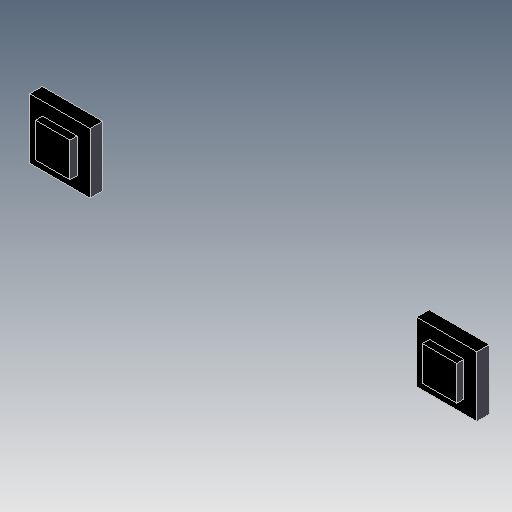
# Autodesk Inventor part: 20210330_5mmFuss_Korpus
Saved by Autodesk Inventor 2021 (Build 250183000, 183)
## iProperties
Created: 2021-03-30
Part Number: 20210330_5mmFuss_Korpus
Material: Acetal Resin, Black
Document SubType Name: Modeling
Designer: Daniel
Density: 1.425 g/cm^3
Appearance: Smooth - Black
Author: Daniel
Autodesk Inventor part; units mm, degrees
ref_plane "YZ Plane" through (0, 0, 0) normal (1, 0, 0) x (0, 1, 0)
ref_plane "XZ Plane" through (0, 0, 0) normal (0, 1, 0) x (-1, 0, 0)
ref_plane "XY Plane" through (0, 0, 0) normal (0, 0, 1) x (1, 0, 0)
sketch "Skizze1" plane through (0, 0, 0) normal (0, 0, 1) x (1, 0, 0)
  line L0 (-89, -12) -> (89, -12)
  line L1 (89, -12) -> (89, 12)
  line L2 (89, 12) -> (-89, 12)
  line L3 (-89, 12) -> (-89, -12)
  line L4 (-89, -12) -> (89, 12) construction
  line L5 (89, -12) -> (-89, 12) construction
  line L6 (65, 12) -> (65, -12)
  line L7 (-65, 12) -> (-65, -12)
  line L8 (-89, 12) -> (-65, -12) construction
  line L9 (-65, 12) -> (-89, -12) construction
  line L10 (89, 12) -> (65, -12) construction
  line L11 (65, 12) -> (89, -12) construction
  point P0 (0, 0)
  dimension "d0" = 178
  dimension "d1" = 24
  dimension "d2" = 24
  dimension "d3" = 24
  constraints: 24 end point, 4 point on line, 2 midpoint, 2 parallel, 2 perpendicular, 1 horizontal, 1 vertical
  measures "d0" distance of L1.end L2.end
  measures "d1" distance of L0.end L1.end
  measures "d2" distance between parallel lines of L1 L6
  measures "d3" distance between parallel lines of L7 L3
extrude "Extrusion1" add sketch "Skizze1" along normal blind 5
sketch "Skizze3" plane through (0, 0, 5) normal (0, 0, 1) x (1, 0, 0)
  line L0 (-89, -12) -> (89, -12)
  line L1 (89, -12) -> (89, 12)
  line L2 (89, 12) -> (-89, 12)
  line L3 (-89, 12) -> (-89, -12)
  line L4 (-89, -12) -> (89, 12) construction
  line L5 (89, -12) -> (-89, 12) construction
  line L6 (65, 12) -> (65, -12)
  line L7 (-65, 12) -> (-65, -12)
  line L8 (-89, 12) -> (-65, -12) construction
  line L9 (-65, 12) -> (-89, -12) construction
  line L10 (89, 12) -> (65, -12) construction
  line L11 (65, 12) -> (89, -12) construction
  line L12 (70.15, -6.85) -> (83.85, -6.85)
  line L13 (83.85, -6.85) -> (83.85, 6.85)
  line L14 (83.85, 6.85) -> (70.15, 6.85)
  line L15 (70.15, 6.85) -> (70.15, -6.85)
  line L16 (70.15, -6.85) -> (83.85, 6.85) construction
  line L17 (83.85, -6.85) -> (70.15, 6.85) construction
  line L18 (-83.85, -6.85) -> (-70.15, -6.85)
  line L19 (-70.15, -6.85) -> (-70.15, 6.85)
  line L20 (-70.15, 6.85) -> (-83.85, 6.85)
  line L21 (-83.85, 6.85) -> (-83.85, -6.85)
  line L22 (-83.85, -6.85) -> (-70.15, 6.85) construction
  line L23 (-70.15, -6.85) -> (-83.85, 6.85) construction
  point P0 (0, 0)
  point P1 (0, 0)
  point P2 (77, 0)
  point P3 (-77, 0)
  dimension "d10" = 178
  dimension "d11" = 24
  dimension "d12" = 24
  dimension "d13" = 24
  dimension "d14" = 13.7
  dimension "d15" = 13.7
  constraints: 48 end point, 8 midpoint, 6 parallel, 6 point on line, 4 perpendicular, 3 horizontal, 1 vertical
  measures "d10" distance of L1.end L2.end
  measures "d11" distance of L0.end L1.end
  measures "d12" distance between parallel lines of L1 L6
  measures "d13" distance between parallel lines of L7 L3
  measures "d14" distance of L13.end L14.end
  measures "d15" distance of L19.end L20.end
extrude "Extrusion2" add sketch "Skizze3" along normal blind 2.85 contours L15 L14 L13 L12 | L21 L20 L19 L18
sketch "Skizze4" plane through (0, 0, 0) normal (0, 0, -1) x (-1, 0, 0)
  line L0 (-89, -12) -> (89, -12)
  line L1 (89, -12) -> (89, 12)
  line L2 (89, 12) -> (-89, 12)
  line L3 (-89, 12) -> (-89, -12)
  line L4 (-89, -12) -> (89, 12) construction
  line L5 (89, -12) -> (-89, 12) construction
  line L6 (65, 12) -> (65, -12)
  line L7 (-65, 12) -> (-65, -12)
  line L8 (-89, 12) -> (-65, -12) construction
  line L9 (-65, 12) -> (-89, -12) construction
  line L10 (89, 12) -> (65, -12) construction
  line L11 (65, 12) -> (89, -12) construction
  line L12 (70, -7) -> (84, -7)
  line L13 (84, -7) -> (84, 7)
  line L14 (84, 7) -> (70, 7)
  line L15 (70, 7) -> (70, -7)
  line L16 (70, -7) -> (84, 7) construction
  line L17 (84, -7) -> (70, 7) construction
  line L18 (-84, -7) -> (-70, -7)
  line L19 (-70, -7) -> (-70, 7)
  line L20 (-70, 7) -> (-84, 7)
  line L21 (-84, 7) -> (-84, -7)
  line L22 (-84, -7) -> (-70, 7) construction
  line L23 (-70, -7) -> (-84, 7) construction
  point P0 (0, 0)
  point P1 (0, 0)
  point P2 (0, 0)
  point P3 (77, 0)
  point P4 (-77, 0)
  dimension "d18" = 178
  dimension "d19" = 24
  dimension "d20" = 24
  dimension "d21" = 24
  dimension "d22" = 14
  dimension "d23" = 14
  constraints: 48 end point, 8 midpoint, 6 parallel, 6 point on line, 4 perpendicular, 3 horizontal, 1 vertical
  measures "d18" distance of L1.end L2.end
  measures "d19" distance of L1.start L1.end
  measures "d20" distance between parallel lines of L1 L6
  measures "d21" distance between parallel lines of L7 L3
  measures "d22" distance of L14.start L14.end
  measures "d23" distance of L19.end L20.end
extrude "Extrusion3" cut sketch "Skizze4" against normal blind 3 contours L15 L14 L13 L12 | L21 L20 L19 L18
sketch "Skizze5" plane through (0, 0, 5) normal (0, 0, 1) x (1, 0, 0)
  line L0 (-89, 12) -> (-89, -12) projected
  line L1 (-89, -12) -> (89, -12) projected
  line L2 (-89, 12) -> (-65, 12)
  line L3 (-65, 12) -> (-65, -12)
  line L4 (-65, -12) -> (-89, -12)
  line L5 (-89, -12) -> (-89, 12)
  line L6 (89, -12) -> (89, 12) projected
  line L7 (89, 12) -> (65, 12)
  line L8 (65, 12) -> (65, -12)
  line L9 (65, -12) -> (89, -12)
  line L10 (89, -12) -> (89, 12)
  line L11 (-65, 12) -> (65, 12)
  line L12 (65, 12) -> (65, -12)
  line L13 (65, -12) -> (-65, -12)
  line L14 (-65, -12) -> (-65, 12)
  point P0 (0, 0)
  point P1 (65, -12)
  dimension "d26" = 24
  dimension "d27" = 24
  constraints: 24 end point, 6 parallel, 3 horizontal, 3 perpendicular, 2 point on line
  measures "d26" distance between parallel lines of L6 L8
  measures "d27" distance between parallel lines of L0 L3
extrude "Extrusion4" cut sketch "Skizze5" against normal through all contours L11 L8 L1 L3
